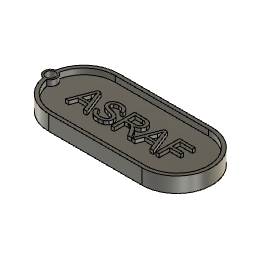
NT (Autodesk Fusion 360 design; units mm, degrees)
Autodesk Fusion 360 part; units mm, degrees
sketch "Sketch1" plane through (0, 0, 0) normal (0, 0, 1) x (1, 0, 0)
  line L0 (20, -15) -> (-20, -15)
  line L1 (-20, 15) -> (20, 15)
  line L2 (35, -15) -> (-35, 15) construction
  line L3 (-35, -15) -> (35, 15) construction
  line L4 (0, 10) -> (0, -10) construction
  arc A0 (20, -15) -> (20, 15) centre (20, 0) ccw
  arc A1 (-20, 15) -> (-20, -15) centre (-20, 0) ccw
  line L5 (-20, -15) -> (20, -15)
  line L6 (20, -13.5) -> (-20, -13.5)
  line L7 (-6, 0) -> (5, 0) construction
  line L8 (20, 13.5) -> (-20, 13.5)
  arc A2 (20, -13.5) -> (20, 13.5) centre (20, 0) ccw
  arc A3 (-20, 13.5) -> (-20, -13.5) centre (-20, 0) ccw
  dimension "d1" = 70
  dimension "d2" = 30
  dimension "d3" = 40
  dimension "d4" = 1.5
  dimension "d5" = 1.5
  constraint horizontal L0
  constraint parallel L0 L1
  constraint coincident L2 origin
  constraint coincident L3 origin
  constraint vertical L4
  constraint horizontal L5
  constraint horizontal L6
  constraint perpendicular L4 L7
  constraint symmetric L6.start L7 L8.start
  constraint symmetric L6.end L7 L8.end
  constraint tangent L6 A2
  constraint symmetric L4 L6.start L6.end
  constraint symmetric L4 L8.start L8.end
  constraint symmetric L4 A2 A3
  measures "d1" distance of L2.end L3.end
  measures "d2" distance of L3.start L2.end
  measures "d3" distance of L0.end L0.start
  measures "d4" distance of L0.end L6.end
  measures "d5" distance of A0 A2
extrude "Extrude1" add sketch "Sketch1" along normal blind 4 contours L0 L1 A0 A1 L5 | L6 L8 A2 A3
extrude "Extrude2" add sketch "Sketch1" along normal blind 6.5
sketch "Sketch2" plane through (0, 0, 0) normal (0, 0, 1) x (1, 0, 0)
  line L0 (-35, 0) -> (-34.25, 0) construction
  circle A0 centre (-34.25, 0) radius 2
  circle A1 centre (-34.25, 0) radius 2.75
  dimension "d10" = 0.75
  dimension "d11" = 4
  dimension "d13" = 5.5
  constraint horizontal L0
  constraint coincident L0.end A0.centre
  constraint concentric A0 A1
  measures "d10" distance of L0.start L0.end
  measures "d11" diameter of A0
  measures "d13" diameter of A1
extrude "Extrude3" cut sketch "Sketch2" along normal blind 14 contours A0 | A1
extrude "Extrude4" add sketch "Sketch2" along normal blind 6.5
sketch "Sketch3" plane through (0, 0, 4) normal (0, 0, 1) x (-1, 0, 0)
  arc A0 (33.2544, 2.5634) -> (33.2544, -2.5634) centre (34.25, 0) ccw
  arc A1 (33.2544, 2.5634) -> (20, 13.5) centre (20, 0) ccw
  line L0 (20, 13.5) -> (-20, 13.5)
  arc A2 (-20, 13.5) -> (-20, -13.5) centre (-20, 0) ccw
  line L1 (-20, -13.5) -> (20, -13.5)
  arc A3 (20, -13.5) -> (33.2544, -2.5634) centre (20, 0) ccw
  line L2 (19.4431, 7.7367) -> (-19.321, 8.0369) construction
  line L3 (-19.321, 8.0369) -> (-19.4431, -7.7367) construction
  line L4 (-19.4431, -7.7367) -> (19.321, -8.0369) construction
  line L5 (19.321, -8.0369) -> (19.4431, 7.7367) construction
  line L6 (19.4431, 7.7367) -> (-19.4431, -7.7367) construction
  line L7 (19.321, -8.0369) -> (-19.321, 8.0369) construction
  dimension "d18" = 10
  text T0 "ASRAF" font "Arial" height 10 align centre middle in box 38.7652 x 15.7741 at (19.4431, 7.7367) x (-0.99997, 0.007746) y (-0.007746, -0.99997) spacing 1
  constraint coincident L2.start
  constraint coincident L3.end
  constraint coincident L4.end
  constraint coincident L2.end
  constraint coincident origin
extrude "Extrude5" add sketch "Sketch3" along normal blind 1.5 text T0
equation "d8 = 4 mm + 2.5 mm"
equation "d10 = ( 1.5 / 2 ) * 1 mm"
